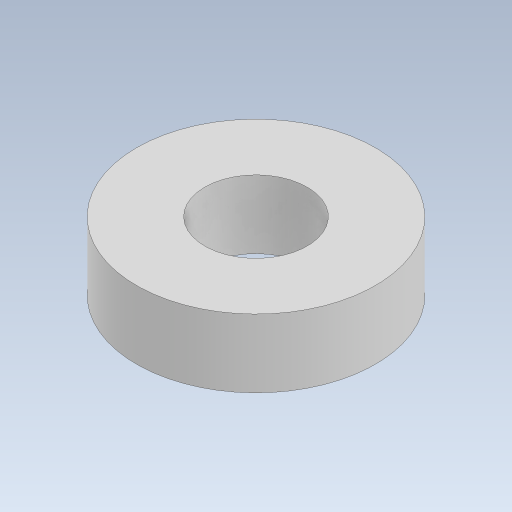
# Autodesk Inventor part: Locker Limit
Saved by Autodesk Inventor 2023.5 (Build 275446000, 446)
## iProperties
Created: 2025-10-05
Part Number: Locker Limit
Material: Generic
Document SubType Name: Modeling
Designer: Guntur
Density: 1 g/cm^3
Appearance: Default
Author: Guntur
## iProperties of the stored document Locker Limit_3DPrint.ipt
Created: 2025-10-05
Part Number: Locker Limit_3DPrint
Material: Generic
Document SubType Name: Modeling
Designer: Guntur
Density: 1 g/cm^3
Appearance: Default
Author: Guntur
Autodesk Inventor part; units mm, degrees
ref_plane "YZ Plane" through (0, 0, 0) normal (1, 0, 0) x (0, 1, 0)
ref_plane "XZ Plane" through (0, 0, 0) normal (0, 1, 0) x (-1, 0, 0)
ref_plane "XY Plane" through (0, 0, 0) normal (0, 0, 1) x (1, 0, 0)
sketch "Sketch1" plane through (0, 0, 0) normal (0, 1, 0) x (-1, 0, 0)
  circle A0 centre (0, 0) radius 1.5
  circle A1 centre (0, 0) radius 3.5
  dimension "d0" = 3
  dimension "d1" = 7
  constraints: 2 centre point, 2 coincident
  measures "d0" diameter of A0
  measures "d1" diameter of A1
extrude "Extrusion1" add sketch "Sketch1" along normal blind 2
body "Solid1"
